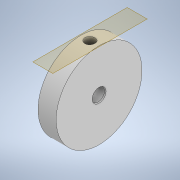
# Autodesk Inventor part: wheel
Saved by Autodesk Inventor 2020 (Build 240168000, 168)
## iProperties
Created: 2020-05-28
Part Number: wheel
Material: Generic
Document SubType Name: Modeling
Designer: Abhinav Roy
Density: 1 g/cm^3
Appearance: Default
Author: Abhinav Roy
Autodesk Inventor part; units mm, degrees
ref_plane "YZ Plane" through (0, 0, 0) normal (1, 0, 0) x (0, 1, 0)
ref_plane "XY Plane" through (0, 0, 0) normal (0, 0, 1) x (1, 0, 0)
sketch "Sketch2" plane through (0, 0, 0) normal (1, 0, 0) x (0, 1, 0)
  circle A0 centre (0, 0) radius 6.4
  circle A1 centre (0, 0) radius 42.5
  dimension "d0" = 12.8
  dimension "d1" = 85
  constraints: 2 centre point, 2 coincident
  measures "d0" diameter of A0
  measures "d1" diameter of A1
extrude "Extrusion1" add sketch "Sketch2" along normal blind 18
ref_plane "Work Plane1" through (0, 42.5, 0) normal (0, 1, 0) x (-1, 0, 0)
sketch "Sketch4" plane through (0, 42.5, 0) normal (0, 1, 0) x (-1, 0, 0)
  circle A0 centre (-9, 0) radius 5
  point P0 (0, 0)
  dimension "d5" = 9
  dimension "d6" = 10
  constraints: 1 centre point
  measures "d5" distance of A0.centre point (0, 0)
  measures "d6" diameter of A0
extrude "Extrusion2" cut sketch "Sketch4" against normal blind 22
sketch "Sketch5" plane through (9, 20.5, 0) normal (0, 1, 0) x (1, 0, 0)
  circle A0 centre (0, 0) radius 2.6
  point P0 (-9, 0)
  dimension "d9" = 5.2
  constraints: 1 centre point
  measures "d9" diameter of A0
extrude "Extrusion3" cut sketch "Sketch5" against normal up to surface round surface about axis through (0, 0, 0) along (1, 0, 0) radius 6.4 far side no
chamfer "Chamfer1" distance 0.5 angle 65 1 edges at (18, -6.4, 0) measured on face at (18, -6.9, 0)
body "Solid1"
